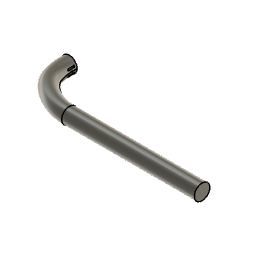
Base1 v7 (Autodesk Fusion 360 archive; units mm, degrees)
design "base pipe"
Autodesk Fusion 360 part; units mm, degrees
note: some values were not read from the file. Set by a fixed rule: which face or edge a step refers to.
sketch "Sketch1" plane through (0, 0, 0) normal (0, 0, 1) x (1, 0, 0)
  line L0 (100, 0) -> (50, 0)
  line L1 (50, 0) -> (20, 30)
  line L2 (20, 30) -> (10, 40)
  line L3 (10, 40) -> (0, 50)
  line L4 (0, 50) -> (0, 100)
  spline S0 degree 5 poles (100, 0) (50, 0) (20, 30) (10, 40) (0, 50) (0, 100) knots 0 0 0 0 0 0 1 1 1 1 1 1
pipe "Pipe1" add diameter 35 path "Sketch1" along S0
sketch "Sketch2" plane through (0, 0, 0) normal (0, 0, 1) x (1, 0, 0)
  line L0 (100, 0) -> (400, 0)
  dimension "d5" = 300
  constraint horizontal L0
  measures "d5" distance of L0.start L0.end
pipe "Pipe2" add diameter 35 path "Sketch2" along L0
sketch "Sketch3" plane through (0, 0, 0) normal (1, 0, 0) x (0, 1, 0)
sketch "Sketch4" plane through (0, 0, 0) normal (1, 0, 0) x (0, 1, 0)
  line L0 (80, -5.1) -> (80, -8.1)
  line L1 (80, -8.1) -> (95.5, -8.1)
  line L2 (95.5, 8.1) -> (80, 8.1)
  line L3 (80, 8.1) -> (80, 5.1)
  line L4 (80, 5.1) -> (95.5, 5.1)
  line L5 (80, -8.1) -> (80, -5.1)
  line L6 (80, -5.1) -> (95.5, -5.1)
  line L7 (80, 8.1) -> (80, 5.1)
  line L8 (80, -5.1) -> (80, -8.1)
  line L9 (95.5, -8.1) -> (95.5, -5.1)
  line L10 (95.5, 5.1) -> (95.5, 8.1)
  circle A0 centre (87.75, -0.0648) radius 1.5
  dimension "d15" = 15.5
  dimension "d16" = 16.2
  dimension "d17" = 3
  dimension "d18" = 3
  dimension "d19" = 3
  constraint vertical L0
  constraint horizontal L1
  constraint vertical L9
  constraint horizontal L2
  constraint vertical L7
  constraint vertical L3
  constraint coincident L4.end L9
  constraint perpendicular L4 L9
  constraint coincident L0.start L7
  constraint perpendicular L6 L9
  constraint collinear L7 L8
  constraint collinear L9 L10
  measures "d15" distance of L0.end L1.end
  measures "d16" distance of L0.end L2.end
  measures "d17" distance of L2.end L3.end
  measures "d18" distance of L0.end L0.start
  measures "d19" diameter of A0
extrude "Extrude1" cut sketch "Sketch4" along normal blind 40
extrude "Extrude2" add 1 faces at (0, 90.3333, 6.1) along direction (1, 0, 0) blind 12.5

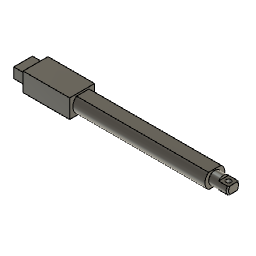
design "LINEAR-ACTUATOR"
Autodesk Fusion 360 part; units mm, degrees
sketch "Sketch1" plane through (0, 0, 0) normal (0, 0, 1) x (1, 0, 0)
  line L0 (0, 0) -> (37.4, 0)
  line L1 (37.4, 0) -> (37.4, 20)
  line L2 (37.4, 20) -> (0, 20)
  line L3 (0, 20) -> (0, 0)
  dimension "d1" = 37.4
  dimension "d2" = 20
  constraint horizontal L0
  constraint vertical L1
  constraint horizontal L2
  constraint vertical L3
  constraint coincident L0.start L3.end
  measures "d1" distance of L0.start L0.end
  measures "d2" distance of L0.start L2.end
extrude "Extrude1" add sketch "Sketch1" along normal blind 15
sketch "Sketch2" plane through (37.4, 0, 0) normal (1, 0, 0) x (0, 1, 0)
  line L0 (0, 0) -> (20, 0)
  line L1 (20, 0) -> (20, 15)
  line L2 (20, 15) -> (0, 15)
  line L3 (0, 15) -> (0, 0)
  line L4 (2.5, 13.5) -> (18.5, 13.5)
  line L5 (18.5, 13.5) -> (18.5, 1.5)
  line L6 (18.5, 1.5) -> (2.5, 1.5)
  line L7 (2.5, 1.5) -> (2.5, 13.5)
  line L8 (2.5, 13.5) -> (5.5, 13.5)
  line L9 (2.5, 1.5) -> (5.5, 1.5)
  arc A0 (5.5, 13.5) -> (5.5, 1.5) centre (10, 7.5) ccw
  line L10 (10.5, 13.5) -> (10.5, 1.5)
  arc A1 (15.5, 1.5) -> (15.5, 13.5) centre (11, 7.5) ccw
  dimension "d5" = 16
  dimension "d6" = 12
  dimension "d7" = 1.5
  dimension "d8" = 1.5
  dimension "d9" = 3
  dimension "d10" = 3
  dimension "d23" = 10
  constraint horizontal L4
  constraint vertical L5
  constraint horizontal L6
  constraint vertical L7
  constraint perpendicular L7 L8
  constraint perpendicular L7 L9
  constraint midpoint L4 L10.start
  constraint midpoint L6 L10.end
  constraint symmetric L8.end L10 A1.end
  constraint symmetric L9.end L10 A1.start
  constraint symmetric A0 L10 A1
  constraint tangent L7 A0
  measures "d5" distance of L4.start L4.end
  measures "d6" distance of L4.start L6.end
  measures "d7" distance of L1 L5
  measures "d8" distance of L2 L4
  measures "d9" distance of L4.start L8.end
  measures "d10" distance of L6.end L9.end
  measures "d23" distance of L8.end A1.end
extrude "Extrude2" add sketch "Sketch2" along normal blind 106 contours L4 L6 A0 L10 | L4 L6 L10 A1
sketch "Sketch3" plane through (0, 0, 0) normal (-1, 0, 0) x (0, -1, 0)
  line L0 (-20, 0) -> (0, 0)
  line L1 (0, 0) -> (0, 15)
  line L2 (0, 15) -> (-20, 15)
  line L3 (-20, 15) -> (-20, 0)
  line L4 (-2.5, 3.5) -> (-17.5, 3.5)
  line L5 (-17.5, 3.5) -> (-17.5, 11.6)
  line L6 (-17.5, 11.6) -> (-2.5, 11.6)
  line L7 (-2.5, 11.6) -> (-2.5, 3.5)
  line L8 (-10, 0) -> (-10, 15)
  line L9 (-20, 7.5) -> (0, 7.5)
  dimension "d13" = 15
  dimension "d14" = 8.1
  dimension "d15" = 4
  dimension "d16" = 7.5
  constraint horizontal L4
  constraint vertical L5
  constraint horizontal L6
  constraint vertical L7
  constraint midpoint L0 L8.start
  constraint midpoint L2 L8.end
  constraint midpoint L3 L9.start
  constraint midpoint L1 L9.end
  measures "d13" distance of L4.start L4.end
  measures "d14" distance of L4.end L5.end
  measures "d15" distance of L4 L9
  measures "d16" distance of L7 L8
extrude "Extrude3" add sketch "Sketch3" along normal blind 10 contours L4 L7 L8 L9 | L4 L5 L8 L9 | L5 L6 L8 L9 | L6 L7 L8 L9
fillet "Fillet1" [suppressed]
fillet "Fillet2" [suppressed]
sketch "Sketch4" plane through (143.4, 0, 0) normal (1, 0, 0) x (0, 1, 0)
  arc A0 (5.5, 13.5) -> (5.5, 1.5) centre (10, 7.5) ccw
  line L0 (5.5, 1.5) -> (15.5, 1.5)
  arc A1 (15.5, 1.5) -> (15.5, 13.5) centre (11, 7.5) ccw
  line L1 (15.5, 13.5) -> (5.5, 13.5)
  line L2 (5.5, 13.5) -> (15.5, 1.5)
  circle A2 centre (10.5, 7.5) radius 5
  dimension "d24" = 10
  constraint coincident A0.start L1.end
  constraint coincident L0.end A1.start
  constraint midpoint L2 A2.centre
  measures "d24" diameter of A2
extrude "Extrude4" add sketch "Sketch4" along normal blind 7 contours L2 A2 | L2 A2
sketch "Sketch5" plane through (150.4, 0, 0) normal (1, 0, 0) x (0, 1, 0)
  circle A0 centre (10.5, 7.5) radius 5
  line L0 (10.5, 7.5) -> (15.5, 7.5)
  line L1 (14.5, 10.5) -> (6.5, 10.5)
  line L2 (14.5, 4.5) -> (6.5, 4.5)
  dimension "d27" = 3
  constraint coincident A0.centre L0.start
  constraint coincident A0 L0.end
  constraint horizontal L0
  constraint coincident A0 L1.start
  constraint coincident A0 L1.end
  constraint horizontal L1
  constraint symmetric L0 L1.start L2.start
  constraint symmetric L0 L1.end L2.end
  measures "d27" distance of L0 L1
extrude "Extrude5" add sketch "Sketch5" along normal blind 8 contours A0 L1 L2
sketch "Sketch6" plane through (0, 0, 4.5) normal (0, 0, -1) x (1, 0, 0)
  line L0 (150.4, -6.5) -> (150.4, -14.5)
  line L1 (150.4, -14.5) -> (158.4, -14.5)
  line L2 (158.4, -14.5) -> (158.4, -6.5)
  line L3 (158.4, -6.5) -> (150.4, -6.5)
  line L4 (158.4, -6.5) -> (150.4, -14.5)
  circle A0 centre (154.4, -10.5) radius 2
  dimension "d30" = 4
  constraint coincident L2.end L3.start
  constraint coincident L0.end L1.start
  constraint midpoint L4 A0.centre
  measures "d30" diameter of A0
extrude "Extrude6" cut sketch "Sketch6" against normal blind 9 contours L4 A0 | L4 A0
fillet "Fillet3" radius 1 2 edges at (158.4, 5.5, 7.5) (158.4, 15.5, 7.5)
equation "d10 = d9"

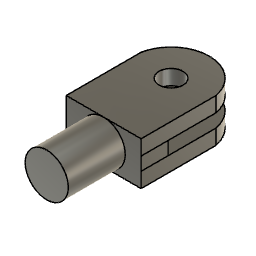
design "lever attach"
Autodesk Fusion 360 part; units mm, degrees
sketch "Sketch1" plane through (0, 0, 0) normal (0, 0, 1) x (1, 0, 0)
  arc A0 (50, 25) -> (25, 25) centre (37.5, 22.5) ccw
  line L0 (0, 0) -> (75, 0)
  circle A1 centre (37.5, 22.5) radius 7.5
  line L1 (25, 25) -> (25, 0)
  line L2 (50, 25) -> (50, 0)
  dimension "d1" = 15
  constraint coincident L0.start origin
  constraint horizontal L0
  constraint concentric A0 A1
  constraint coincident L0 L1.end
  constraint perpendicular L0 L1
  constraint coincident L0 L2.end
  constraint perpendicular L0 L2
  measures "d1" diameter of A1
extrude "Extrude1" add sketch "Sketch1" along normal blind 5 makes body 1
copy_body "CopyPasteBodies1" bodies 1 makes body 2
move_body "Move1" bodies 2 to x (1, 0, 0) y (0, 1, 0) z (0, 0, 1) at (0, 0, 9.4)
sketch "Sketch2" plane through (0, 0, 0) normal (0, -1, 0) x (1, 0, 0)
  line L0 (25, 9.4) -> (50, 9.4)
  line L1 (50, 9.4) -> (50, 14.4)
  line L2 (50, 14.4) -> (25, 14.4)
  line L3 (25, 14.4) -> (25, 9.4)
  line L4 (25, 5) -> (25, 9.4)
  line L5 (50, 5) -> (50, 9.4)
  line L6 (25, 5) -> (50, 5)
  line L7 (50, 9.4) -> (25, 9.4)
  constraint coincident L0.start L3.end
  constraint coincident L0.end L1.start
  constraint parallel L0 L6
extrude "Extrude2" add sketch "Sketch2" against normal blind 9 contours L0 L4 L5 L6 L7 bodies 1 2
sketch "Sketch3" plane through (0, 0, 0) normal (0, -1, 0) x (1, 0, 0)
  line L0 (25, 0) -> (50, 0)
  line L1 (50, 0) -> (50, 5)
  line L2 (50, 5) -> (50, 9.4)
  line L3 (50, 9.4) -> (50, 14.4)
  line L4 (50, 14.4) -> (25, 14.4)
  line L5 (25, 14.4) -> (25, 9.4)
  line L6 (25, 9.4) -> (25, 5)
  line L7 (25, 5) -> (25, 0)
  circle A0 centre (37.5, 7.2) radius 7.2
  constraint tangent L0 A0
extrude "Extrude3" add sketch "Sketch3" along normal blind 19 contours A0 bodies 1
move_face "OffsetFaces1" offset 3.5 1 faces at (44.9907, 22.1262, 12.7333) on bodies 1
move_face "OffsetFaces2" offset 3.5 1 faces at (44.9907, 22.1262, 3.3333) on bodies 1

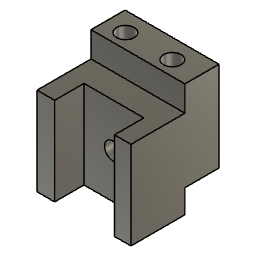
design "Midconnector"
Autodesk Fusion 360 part; units mm, degrees
sketch "Sketch1" plane through (0, 0, 0) normal (0, 0, 1) x (1, 0, 0)
  line L0 (16, 0) -> (16, 15)
  line L1 (16, 15) -> (0, 15)
  line L2 (0, 15) -> (0, 0)
  line L3 (0, 0) -> (3, 0)
  line L4 (3, 0) -> (3, 5)
  line L5 (3, 5) -> (13.2, 5)
  line L6 (13.2, 5) -> (13.2, 0)
  line L7 (0, 0) -> (3, 0)
  line L8 (13.2, 0) -> (16, 0)
  dimension "d1" = 16
  dimension "d2" = 15
  dimension "d3" = 5
  dimension "d4" = 10.2
  constraint horizontal L7
  constraint vertical L0
  constraint horizontal L1
  constraint vertical L2
  constraint coincident L2.end L3.start
  constraint perpendicular L4 L7
  constraint perpendicular L4 L5
  constraint coincident L6.end L7
  constraint perpendicular L6 L7
  constraint collinear L7 L8
  measures "d1" distance of L2.end L0.start
  measures "d2" distance of L2.end L1.end
  measures "d3" distance of L3.end L4.end
  measures "d4" distance of L4.end L5.end
extrude "Extrude1" add sketch "Sketch1" along normal blind 15
sketch "Sketch2" plane through (0, 5, 0) normal (0, -1, 0) x (1, 0, 0)
  line L0 (3, 0) -> (13.2, 0)
  line L1 (13.2, 0) -> (13.2, 15)
  line L2 (13.2, 15) -> (3, 15)
  line L3 (3, 15) -> (3, 0)
  line L4 (0, 0) -> (3, 0)
  line L5 (8, 6) -> (8, 7.5)
  circle A0 centre (8, 7.5) radius 1.5
  dimension "d9" = 3
  constraint coincident L4.start origin
  constraint parallel L0 L4
  constraint perpendicular L4 L5
  constraint coincident L5.end A0.centre
  constraint coincident A0 L5.start
  measures "d9" diameter of A0
extrude "Extrude2" cut sketch "Sketch2" against normal blind 19 contours A0
sketch "Sketch3" plane through (0, 15, 0) normal (0, 1, 0) x (-1, 0, 0)
  circle A0 centre (-8, 7.5) radius 1.5
  line L0 (-16, 0) -> (0, 0)
  line L1 (0, 0) -> (0, 15)
  line L2 (0, 15) -> (-16, 15)
  line L3 (-16, 15) -> (-16, 0)
  line L4 (0, 0) -> (0, 4)
  line L5 (0, 4) -> (-16, 4)
  line L6 (0, 15) -> (0, 11)
  line L7 (0, 11) -> (-16, 11)
  dimension "d12" = 4
  dimension "d13" = 4
  constraint coincident L0.end L1.start
  constraint perpendicular L0 L4
  constraint coincident L3 L5.end
  constraint perpendicular L3 L5
  constraint coincident L1.end L2.start
  constraint perpendicular L2 L6
  constraint coincident L3 L7.end
  constraint perpendicular L3 L7
  measures "d12" distance of L0.end L4.end
  measures "d13" distance of L1.end L6.end
extrude "Extrude3" cut sketch "Sketch3" against normal blind 5.8 contours L0 L1 L3 L4 L5 | L1 L2 L3 L6 L7
sketch "Sketch4" plane through (0, 0, 11) normal (0, 0, 1) x (-1, 0, 0)
  line L0 (-16, -15) -> (0, -15)
  line L1 (0, -15) -> (0, -9.2)
  line L2 (0, -9.2) -> (-16, -9.2)
  line L3 (-16, -9.2) -> (-16, -15)
  line L4 (-12.85, -11.7) -> (-11.35, -11.7)
  circle A0 centre (-11.35, -11.7) radius 1.5
  circle A1 centre (-3.35, -11.7) radius 1.5
  line L5 (-11.35, -11.7) -> (-9.85, -11.7)
  line L6 (-4.85, -11.7) -> (-3.35, -11.7)
  dimension "d18" = 3
  dimension "d19" = 8
  dimension "d20" = 3
  constraint coincident L4.end A0.centre
  constraint parallel L4 L5
  constraint coincident A1.centre L6.end
  constraint coincident A0 L5.end
  constraint coincident A1 L6.start
  constraint collinear L5 L6
  constraint coincident A0 L4.start
  measures "d18" diameter of A0
  measures "d19" distance of L4.end A1.centre
  measures "d20" diameter of A1
extrude "Extrude4" cut sketch "Sketch4" against normal blind 2 contours L4 A0 L5 | L4 A0 L5 | A1
sketch "Sketch5" plane through (0, 0, 4) normal (0, 0, -1) x (1, 0, 0)
  line L0 (0, -15) -> (16, -15)
  line L1 (16, -15) -> (16, -9.2)
  line L2 (16, -9.2) -> (0, -9.2)
  line L3 (0, -9.2) -> (0, -15)
  circle A0 centre (4.65, -11.7) radius 1.5
  circle A1 centre (12.65, -11.7) radius 1.5
  line L4 (11.15, -11.7) -> (12.65, -11.7)
  dimension "d25" = 3
  dimension "d26" = 8
  dimension "d27" = 3
  constraint coincident A1.centre L4.end
  constraint coincident A1 L4.start
  measures "d25" diameter of A0
  measures "d26" distance of A0.centre A1.centre
  measures "d27" diameter of A1
extrude "Extrude5" cut sketch "Sketch5" against normal blind 2 contours A0 | A1
move_face "OffsetFaces1" offset 8.325 1 faces at (14.9444, 12.0412, 11)

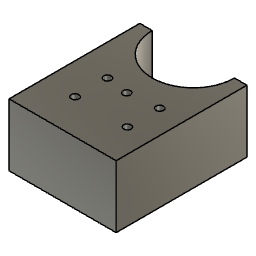
design "Torch holder connector1"
Autodesk Fusion 360 part; units mm, degrees
sketch "Sketch1" plane through (0, 0, 0) normal (0, 0, 1) x (1, 0, 0)
  line L0 (0, 0) -> (43, 0)
  line L1 (43, 0) -> (43, 52.5)
  line L2 (0, 52.5) -> (0, 0)
  arc A0 (5, 52.5) -> (38, 52.5) centre (21.5, 52.5) ccw
  line L3 (43, 52.5) -> (38, 52.5)
  line L4 (5, 52.5) -> (0, 52.5)
  line L5 (11, 14) -> (12.5, 14)
  circle A1 centre (12.5, 14) radius 1.5
  circle A2 centre (33.5, 14) radius 1.5
  circle A3 centre (12.5, 27) radius 1.5
  circle A4 centre (33.5, 27) radius 1.5
  line L6 (33.5, 14) -> (33.5, 15.5)
  line L7 (33.5, 25.5) -> (33.5, 27)
  line L8 (12.5, 14) -> (14, 14)
  line L9 (32, 14) -> (33.5, 14)
  line L10 (12.5, 14) -> (12.5, 15.5)
  line L11 (12.5, 25.5) -> (12.5, 27)
  line L12 (21.5, 28.25) -> (21.5, 26.75)
  line L13 (21.5, 0) -> (21.5, 25.75)
  circle A5 centre (21.5, 25.75) radius 1.5
  dimension "d1" = 43
  dimension "d2" = 52.5
  dimension "d6" = 3
  dimension "d7" = 21
  dimension "d8" = 3
  dimension "d9" = 13
  dimension "d10" = 3
  dimension "d11" = 13
  dimension "d12" = 3
  dimension "d15" = 25.75
  dimension "d16" = 3
  constraint horizontal L0
  constraint vertical L1
  constraint horizontal L3
  constraint vertical L2
  constraint coincident L0.start L2.end
  constraint coincident A0.start L3
  constraint collinear L3 L4
  constraint coincident A0.centre L3
  constraint coincident L5.end A1.centre
  constraint coincident A1 L5.start
  constraint parallel L5 L8
  constraint coincident A2.centre L6.start
  constraint perpendicular L5 L10
  constraint coincident A3.centre L11.end
  constraint perpendicular L6 L8
  constraint coincident A4.centre L7.end
  constraint coincident A2 L6.end
  constraint coincident A4 L7.start
  constraint collinear L6 L7
  constraint coincident A1 L8.end
  constraint coincident A2 L9.start
  constraint collinear L8 L9
  constraint coincident A1 L10.end
  constraint coincident A3 L11.start
  constraint collinear L10 L11
  constraint vertical L12
  constraint midpoint L0 L13.start
  constraint perpendicular L0 L13
  constraint coincident L13.end A5.centre
  measures "d1" distance of L0.start L0.end
  measures "d2" distance of L0.start L2.start
  measures "d6" diameter of A1
  measures "d7" distance of L5.end A2.centre
  measures "d8" diameter of A2
  measures "d9" distance of L5.end A3.centre
  measures "d10" diameter of A3
  measures "d11" distance of A2.centre A4.centre
  measures "d12" diameter of A4
  measures "d15" distance of L13.start L13.end
  measures "d16" diameter of A5
extrude "Extrude1" add sketch "Sketch1" along normal blind 25

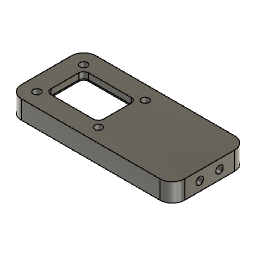
design "ACTUATOR-SLIDER-TOP-CONNECTOR"
Autodesk Fusion 360 part; units mm, degrees
sketch "Sketch1" plane through (0, 0, 0) normal (0, 0, 1) x (1, 0, 0)
  line L0 (2, 0) -> (28.3, 0)
  line L1 (30.3, 2) -> (30.3, 22.3)
  line L2 (28.3, 24.3) -> (2, 24.3)
  line L3 (0, 22.3) -> (0, 2)
  arc A0 (0, 2) -> (2, 0) centre (2, 2) ccw
  arc A1 (2, 24.3) -> (0, 22.3) centre (2, 22.3) ccw
  arc A2 (30.3, 22.3) -> (28.3, 24.3) centre (28.3, 22.3) ccw
  arc A3 (28.3, 0) -> (30.3, 2) centre (28.3, 2) ccw
  line L4 (-3, 22.3) -> (-3, 2)
  arc A4 (-3, 2) -> (2, -3) centre (2, 2) ccw
  line L5 (2, -3) -> (28.3, -3)
  arc A5 (28.3, -3) -> (33.3, 2) centre (28.3, 2) ccw
  line L6 (33.3, 2) -> (33.3, 22.3)
  arc A6 (33.3, 22.3) -> (28.3, 27.3) centre (28.3, 22.3) ccw
  line L7 (28.3, 27.3) -> (2, 27.3)
  arc A7 (2, 27.3) -> (-3, 22.3) centre (2, 22.3) ccw
  line L8 (28.3, -3) -> (53.3, -3)
  line L9 (58.3, 2) -> (58.3, 22.3)
  line L10 (53.3, 27.3) -> (28.3, 27.3)
  line L11 (28.3, 27.3) -> (28.3, -3)
  arc A8 (58.3, 22.3) -> (53.3, 27.3) centre (53.3, 22.3) ccw
  arc A9 (53.3, -3) -> (58.3, 2) centre (53.3, 2) ccw
  point P0 (30.3, 0)
  point P1 (0, 24.3)
  point P2 (58.3, -3)
  dimension "d1" = 30.3
  dimension "d2" = 24.3
  dimension "d3" = 2
  dimension "d4" = 3
  dimension "d40" = 30
  dimension "d76" = 5
  dimension "d77" = 5
  constraint horizontal L0
  constraint vertical L1
  constraint horizontal L2
  constraint vertical L3
  constraint coincident origin L3
  constraint coincident origin L0
  constraint tangent L3 A0
  constraint tangent L0 A0
  constraint coincident P1 L3
  constraint coincident P1 L2
  constraint tangent L3 A1
  constraint tangent L2 A1
  constraint equal A0 A1
  constraint tangent L2 A2
  constraint tangent L1 A2
  constraint equal A0 A2
  constraint coincident P0 L1
  constraint coincident P0 L0
  constraint tangent L1 A3
  constraint tangent L0 A3
  constraint equal A0 A3
  constraint horizontal L8
  constraint vertical L9
  constraint horizontal L10
  constraint vertical L11
  constraint tangent L9 A8
  constraint tangent L10 A8
  constraint coincident P2 L8
  constraint coincident P2 L9
  constraint tangent L8 A9
  constraint tangent L9 A9
  measures "d1" distance of origin P0
  measures "d2" distance of origin P1
  measures "d3" radius of A0
  measures "d40" distance of L5.end P2
  measures "d76" radius of A8
  measures "d77" radius of A9
extrude "Extrude1" add sketch "Sketch1" along normal blind 5 contours L0 L2 L3 A0 A1 L4 A4 L5 L7 A7 L11 | L1 A2 A3 A5 L6 A6 L11
sketch "Sketch2" plane through (0, 0, 5) normal (0, 0, 1) x (-1, 0, 0)
  arc A0 (-28.3, 0) -> (-30.3, -2) centre (-28.3, -2) ccw
  line L0 (-28.3, 0) -> (-2, 0)
  arc A1 (0, -2) -> (-2, 0) centre (-2, -2) ccw
  line L1 (0, -2) -> (0, -22.3)
  arc A2 (-2, -24.3) -> (0, -22.3) centre (-2, -22.3) ccw
  line L2 (-2, -24.3) -> (-28.3, -24.3)
  arc A3 (-30.3, -22.3) -> (-28.3, -24.3) centre (-28.3, -22.3) ccw
  line L3 (-30.3, -22.3) -> (-30.3, -2)
  arc A4 (-2, -27.3) -> (3, -22.3) centre (-2, -22.3) ccw
  line L4 (3, -22.3) -> (3, -2)
  arc A5 (3, -2) -> (-2, 3) centre (-2, -2) ccw
  line L5 (-2, 3) -> (-28.3, 3)
  arc A6 (-28.3, 3) -> (-33.3, -2) centre (-28.3, -2) ccw
  line L6 (-33.3, -2) -> (-33.3, -22.3)
  arc A7 (-33.3, -22.3) -> (-28.3, -27.3) centre (-28.3, -22.3) ccw
  line L7 (-28.3, -27.3) -> (-2, -27.3)
  line L8 (-28.3, 3) -> (-58.3, 3)
  line L9 (-63.3, -2) -> (-63.3, -22.3)
  line L10 (-58.3, -27.3) -> (-28.3, -27.3)
  line L11 (-28.3, -27.3) -> (-28.3, 3)
  line L12 (-15.15, 3) -> (-15.15, -27.3)
  line L13 (3, -12.15) -> (-33.3, -12.15)
  line L14 (-2.65, -2.65) -> (-27.65, -2.65)
  line L15 (-27.65, -2.65) -> (-27.65, -21.65)
  line L16 (-27.65, -21.65) -> (-2.65, -21.65)
  line L17 (-2.65, -21.65) -> (-2.65, -2.65)
  line L18 (-15.15, -2.65) -> (-15.15, -21.65)
  line L19 (-2.65, -12.15) -> (-27.65, -12.15)
  circle A8 centre (-2.65, -2.65) radius 1.5
  circle A9 centre (-27.65, -2.65) radius 1.5
  circle A10 centre (-2.65, -21.65) radius 1.5
  circle A11 centre (-27.65, -21.65) radius 1.5
  line L20 (-23.8, -4.5) -> (-6.5, -4.5)
  line L21 (-25.8, -17.8) -> (-25.8, -6.5)
  line L22 (-6.5, -19.8) -> (-23.8, -19.8)
  line L23 (-4.5, -6.5) -> (-4.5, -17.8)
  arc A12 (-4.5, -6.5) -> (-6.5, -4.5) centre (-6.5, -6.5) ccw
  arc A13 (-23.8, -4.5) -> (-25.8, -6.5) centre (-23.8, -6.5) ccw
  arc A14 (-25.8, -17.8) -> (-23.8, -19.8) centre (-23.8, -17.8) ccw
  arc A15 (-6.5, -19.8) -> (-4.5, -17.8) centre (-6.5, -17.8) ccw
  arc A16 (-63.3, -22.3) -> (-58.3, -27.3) centre (-58.3, -22.3) ccw
  arc A17 (-58.3, 3) -> (-63.3, -2) centre (-58.3, -2) ccw
  point P0 (-63.3, 3)
  dimension "d9" = 35
  dimension "d34" = 25
  dimension "d35" = 19
  dimension "d36" = 3
  dimension "d37" = 3
  dimension "d38" = 3
  dimension "d39" = 3
  dimension "d54" = 2
  dimension "d75" = 0.65
  dimension "d78" = 5
  constraint horizontal L8
  constraint vertical L9
  constraint horizontal L10
  constraint vertical L11
  constraint coincident L5.end A6.start
  constraint coincident A7.end L7.start
  constraint midpoint L5 L12.start
  constraint midpoint L7 L12.end
  constraint midpoint L4 L13.start
  constraint midpoint L6 L13.end
  constraint horizontal L14
  constraint vertical L15
  constraint horizontal L16
  constraint vertical L17
  constraint midpoint L14 L18.start
  constraint midpoint L16 L18.end
  constraint midpoint L17 L19.start
  constraint midpoint L15 L19.end
  constraint collinear L12 L18
  constraint collinear L13 L19
  constraint coincident L14.start L17.end
  constraint coincident L14.end L15.start
  constraint coincident L16.end L17.start
  constraint coincident L15.end L16.start
  constraint parallel L0 L20
  constraint parallel L3 L21
  constraint parallel L2 L22
  constraint parallel L1 L23
  constraint tangent L20 A12
  constraint tangent L23 A12
  constraint tangent L20 A13
  constraint tangent L21 A13
  constraint equal A12 A13
  constraint tangent L21 A14
  constraint tangent L22 A14
  constraint equal A12 A14
  constraint tangent L22 A15
  constraint tangent L23 A15
  constraint equal A12 A15
  constraint tangent L10 A16
  constraint tangent L9 A16
  constraint coincident P0 L9
  constraint coincident P0 L8
  constraint tangent L9 A17
  constraint tangent L8 A17
  constraint equal A16 A17
  measures "d9" distance of L5.end P0
  measures "d34" distance of L14.start L14.end
  measures "d35" distance of L14.start L16.end
  measures "d36" diameter of A8
  measures "d37" diameter of A9
  measures "d38" diameter of A10
  measures "d39" diameter of A11
  measures "d54" radius of A12
  measures "d75" distance of L11 L15.end
  measures "d78" radius of A16
extrude "Extrude2" add sketch "Sketch2" along normal blind 2.5 contours A0 L3 L11 L13 A9 | L0 L5 L11 L12 | A0 L3 A6 L6 L11 L13 | L0 L11 L12 L14 A9 | L0 A1 L1 L4 A5 L5 L12 L13 | L0 A1 L1 L12 L13 L14 L17 A8 | A6 L6 A7 L8 L9 L10 A16 A17 | A3 L3 L11 L13 A11 | A3 L3 L6 A7 L11 L13 | L12 L13 L14 L17 L18 L19 A8 L20 L23 A12 | L12 L13 L14 L15 L18 L19 A9 L20 L21 A13 | L11 L13 L15 A9 | L11 L13 L15 A11 | L2 L11 L12 L16 A11 | L2 L7 L11 L12 | L12 L13 L15 L16 L18 L19 A11 L21 L22 A14 | L1 A2 L2 A4 L4 L7 L12 L13 | L1 A2 L2 L12 L13 L16 L17 A10 | L12 L13 L16 L17 L18 L19 A10 L22 L23 A15
sketch "Sketch3" plane through (0, 0, 5) normal (0, 0, -1) x (1, 0, 0)
  arc A0 (28.3, -27.3) -> (33.3, -22.3) centre (28.3, -22.3) ccw
  line L0 (28.3, -27.3) -> (58.3, -27.3)
  line L1 (63.3, -22.3) -> (63.3, -2)
  line L2 (58.3, 3) -> (28.3, 3)
  arc A1 (33.3, -2) -> (28.3, 3) centre (28.3, -2) ccw
  line L3 (33.3, -2) -> (33.3, -22.3)
  line L4 (58.3, -27.3) -> (53.3, -27.3)
  line L5 (53.3, -27.3) -> (53.3, 7)
  line L6 (53.3, 7) -> (58.3, 7)
  line L7 (58.3, 7) -> (58.3, -27.3)
  arc A2 (58.3, -27.3) -> (63.3, -22.3) centre (58.3, -22.3) ccw
  arc A3 (63.3, -2) -> (58.3, 3) centre (58.3, -2) ccw
  dimension "d10" = 5
  constraint horizontal L4
  constraint vertical L5
  constraint horizontal L6
  constraint vertical L7
  constraint coincident L0.end L4.start
  measures "d10" distance of L0.end L4.end
extrude "Extrude3" add sketch "Sketch3" along normal blind 5 contours A0 L0 L2 A1 L3 L5 | L0 L2 L4 L5 L7 | L1 L7 A2 A3
sketch "Sketch4" plane through (63.3, 0, 0) normal (1, 0, 0) x (0, 1, 0)
  line L0 (2, 0) -> (22.3, 0)
  line L1 (2, 0) -> (22.3, 0)
  line L2 (22.3, 0) -> (22.3, 7.5)
  line L3 (22.3, 7.5) -> (2, 7.5)
  line L4 (2, 7.5) -> (2, 0)
  line L5 (2, 3.75) -> (22.3, 3.75)
  circle A0 centre (8.15, 3.75) radius 1.5
  line L6 (12.15, 7.5) -> (12.15, 0)
  circle A1 centre (16.15, 3.75) radius 1.5
  line L7 (22.3, 0) -> (22.3, 7.5)
  line L8 (22.3, 7.5) -> (2, 7.5)
  line L9 (2, 7.5) -> (2, 0)
  dimension "d14" = 3
  dimension "d15" = 4
  constraint horizontal L1
  constraint vertical L2
  constraint horizontal L3
  constraint vertical L4
  constraint coincident L0.start L1.start
  constraint midpoint L4 L5.start
  constraint midpoint L2 L5.end
  constraint coincident L5 A0.centre
  constraint midpoint L3 L6.start
  constraint midpoint L0 L6.end
  constraint symmetric A0 L6 A1
  measures "d14" diameter of A0
  measures "d15" distance of A0.centre L6
extrude "Extrude4" cut sketch "Sketch4" against normal blind 20 contours L5 A0 | L5 A0 | L5 A1 | L5 A1
fillet "Fillet3" [rolled back] radius 7
sketch "Sketch5" plane through (0, 0, 7.5) normal (0, 0, 1) x (-1, 0, 0)
  arc A0 (-66.3, 7) -> (-73.3, 0) centre (-66.3, 0) ccw
  line L0 (-73.3, 0) -> (-73.3, -24.3)
  arc A1 (-73.3, -24.3) -> (-66.3, -31.3) centre (-66.3, -24.3) ccw
  line L1 (-66.3, -31.3) -> (-2, -31.3)
  arc A2 (-2, -31.3) -> (7, -22.3) centre (-2, -22.3) ccw
  line L2 (7, -22.3) -> (7, -2)
  arc A3 (7, -2) -> (-2, 7) centre (-2, -2) ccw
  line L3 (-2, 7) -> (-66.3, 7)
  circle A4 centre (-27.65, -2.65) radius 1.5
  circle A5 centre (-2.65, -2.65) radius 1.5
  circle A6 centre (-27.65, -21.65) radius 1.5
  circle A7 centre (-2.65, -21.65) radius 1.5
  line L4 (-63, -27.3) -> (-68.3, -27.3)
  line L5 (-68.3, -27.3) -> (-68.3, 3)
  line L6 (-68.3, 3) -> (-63, 3)
  line L7 (-63, 3) -> (-63, -27.3)
  line L8 (-73.3, -12.15) -> (7, -12.15)
  line L9 (-63, -12.15) -> (-68.3, -12.15)
  arc A8 (-25.8, -17.8) -> (-23.8, -19.8) centre (-23.8, -17.8) ccw
  line L10 (-25.8, -17.8) -> (-25.8, -6.5)
  arc A9 (-23.8, -4.5) -> (-25.8, -6.5) centre (-23.8, -6.5) ccw
  line L11 (-23.8, -4.5) -> (-6.5, -4.5)
  arc A10 (-4.5, -6.5) -> (-6.5, -4.5) centre (-6.5, -6.5) ccw
  line L12 (-4.5, -6.5) -> (-4.5, -17.8)
  arc A11 (-6.5, -19.8) -> (-4.5, -17.8) centre (-6.5, -17.8) ccw
  line L13 (-6.5, -19.8) -> (-23.8, -19.8)
  dimension "d48" = 5.3
  dimension "d49" = 30.3
  dimension "d50" = 5
  constraint horizontal L4
  constraint vertical L5
  constraint horizontal L6
  constraint vertical L7
  constraint midpoint L0 L8.start
  constraint midpoint L2 L8.end
  constraint midpoint L7 L9.start
  constraint midpoint L5 L9.end
  constraint collinear L8 L9
  measures "d48" distance of L4.start L4.end
  measures "d49" distance of L4.start L6.end
  measures "d50" distance of L0 L5
extrude "Extrude5" [rolled back] along distance -7.5 taper angle 0
fillet "Fillet4" [rolled back] radius 2.5
ref_plane "WorkPlane1" through (33.15, 12.15, -2.5) normal (0, 0, -1) x (-1, 0, 0)
mirror "Mirror1" [rolled back] mirror stitch tolerance 0.1
sketch "Sketch6" plane through (0, 0, -10) normal (0, 0, 1) x (-1, 0, 0)
  line L0 (-30.3, -2) -> (-30.3, -22.3)
  arc A0 (-30.3, -22.3) -> (-28.3, -24.3) centre (-28.3, -22.3) ccw
  line L1 (-28.3, -24.3) -> (-2, -24.3)
  arc A1 (-2, -24.3) -> (0, -22.3) centre (-2, -22.3) ccw
  line L2 (0, -22.3) -> (0, -2)
  arc A2 (0, -2) -> (-2, 0) centre (-2, -2) ccw
  line L3 (-2, 0) -> (-28.3, 0)
  arc A3 (-28.3, 0) -> (-30.3, -2) centre (-28.3, -2) ccw
  circle A4 centre (-27.65, -21.65) radius 1.5
  circle A5 centre (-2.65, -21.65) radius 1.5
  circle A6 centre (-27.65, -2.65) radius 1.5
  arc A7 (-25.8, -17.8) -> (-23.8, -19.8) centre (-23.8, -17.8) ccw
  line L4 (-25.8, -17.8) -> (-25.8, -6.5)
  arc A8 (-23.8, -4.5) -> (-25.8, -6.5) centre (-23.8, -6.5) ccw
  line L5 (-23.8, -4.5) -> (-6.5, -4.5)
  arc A9 (-4.5, -6.5) -> (-6.5, -4.5) centre (-6.5, -6.5) ccw
  line L6 (-4.5, -6.5) -> (-4.5, -17.8)
  arc A10 (-6.5, -19.8) -> (-4.5, -17.8) centre (-6.5, -17.8) ccw
  line L7 (-6.5, -19.8) -> (-23.8, -19.8)
  circle A11 centre (-2.65, -2.65) radius 1.5
extrude "Extrude6" [rolled back] along distance -2.5 taper angle 0
sketch "Sketch8" plane through (0, 0, -5) normal (0, 0, 1) x (-1, 0, 0)
  line L0 (-68.3, -24.8) -> (-68.3, 0.5)
  arc A0 (-65.8, 3) -> (-68.3, 0.5) centre (-65.8, 0.5) ccw
  line L1 (-65.8, 3) -> (-65.5, 3)
  arc A1 (-63, 0.5) -> (-65.5, 3) centre (-65.5, 0.5) ccw
  line L2 (-63, 0.5) -> (-63, -24.8)
  arc A2 (-65.5, -27.3) -> (-63, -24.8) centre (-65.5, -24.8) ccw
  line L3 (-65.5, -27.3) -> (-65.8, -27.3)
  arc A3 (-68.3, -24.8) -> (-65.8, -27.3) centre (-65.8, -24.8) ccw
  arc A4 (-28.3, 0) -> (-30.3, -2) centre (-28.3, -2) ccw
  line L4 (-28.3, 0) -> (-2, 0)
  arc A5 (0, -2) -> (-2, 0) centre (-2, -2) ccw
  line L5 (0, -2) -> (0, -22.3)
  arc A6 (-2, -24.3) -> (0, -22.3) centre (-2, -22.3) ccw
  line L6 (-2, -24.3) -> (-28.3, -24.3)
  arc A7 (-30.3, -22.3) -> (-28.3, -24.3) centre (-28.3, -22.3) ccw
  line L7 (-30.3, -22.3) -> (-30.3, -2)
  arc A8 (-66.3, 7) -> (-73.3, 0) centre (-66.3, 0) ccw
  line L8 (-73.3, 0) -> (-73.3, -24.3)
  arc A9 (-73.3, -24.3) -> (-66.3, -31.3) centre (-66.3, -24.3) ccw
  line L9 (-66.3, -31.3) -> (-2, -31.3)
  arc A10 (-2, -31.3) -> (7, -22.3) centre (-2, -22.3) ccw
  line L10 (7, -22.3) -> (7, -2)
  arc A11 (7, -2) -> (-2, 7) centre (-2, -2) ccw
  line L11 (-2, 7) -> (-66.3, 7)
  line L12 (-71.3, 0) -> (-71.3, -24.3)
  arc A12 (-71.3, -24.3) -> (-66.3, -29.3) centre (-66.3, -24.3) ccw
  line L13 (-66.3, -29.3) -> (-2, -29.3)
  arc A13 (-2, -29.3) -> (5, -22.3) centre (-2, -22.3) ccw
  line L14 (5, -22.3) -> (5, -2)
  arc A14 (5, -2) -> (-2, 5) centre (-2, -2) ccw
  line L15 (-2, 5) -> (-66.3, 5)
  arc A15 (-66.3, 5) -> (-71.3, 0) centre (-66.3, 0) ccw
  arc A16 (-32.3, -22.3) -> (-28.3, -26.3) centre (-28.3, -22.3) ccw
  line L16 (-2, -26.3) -> (-28.3, -26.3)
  arc A17 (-2, -26.3) -> (2, -22.3) centre (-2, -22.3) ccw
  line L17 (2, -2) -> (2, -22.3)
  arc A18 (2, -2) -> (-2, 2) centre (-2, -2) ccw
  line L18 (-28.3, 2) -> (-2, 2)
  arc A19 (-28.3, 2) -> (-32.3, -2) centre (-28.3, -2) ccw
  line L19 (-32.3, -22.3) -> (-32.3, -2)
  line L20 (-65.8, 4) -> (-65.5, 4)
  arc A20 (-62, 0.5) -> (-65.5, 4) centre (-65.5, 0.5) ccw
  line L21 (-62, 0.5) -> (-62, -24.8)
  arc A21 (-65.5, -28.3) -> (-62, -24.8) centre (-65.5, -24.8) ccw
  line L22 (-65.5, -28.3) -> (-65.8, -28.3)
  arc A22 (-69.3, -24.8) -> (-65.8, -28.3) centre (-65.8, -24.8) ccw
  line L23 (-69.3, -24.8) -> (-69.3, 0.5)
  arc A23 (-65.8, 4) -> (-69.3, 0.5) centre (-65.8, 0.5) ccw
  dimension "d70" = -2
  dimension "d73" = -2
  dimension "d74" = 1
  measures "d73" distance of A7
extrude "Extrude8" [rolled back] side1offset 0 taper angle 0
sketch "Sketch7" plane through (0, 0, -10) normal (0, 0, 1) x (-1, 0, 0)
  line L0 (-53.3, -24.8) -> (-53.3, 0.5)
  arc A0 (-50.8, 3) -> (-53.3, 0.5) centre (-50.8, 0.5) ccw
  line L1 (-50.8, 3) -> (-50.5, 3)
  arc A1 (-48, 0.5) -> (-50.5, 3) centre (-50.5, 0.5) ccw
  line L2 (-48, 0.5) -> (-48, -24.8)
  arc A2 (-50.5, -27.3) -> (-48, -24.8) centre (-50.5, -24.8) ccw
  line L3 (-50.5, -27.3) -> (-50.8, -27.3)
  arc A3 (-53.3, -24.8) -> (-50.8, -27.3) centre (-50.8, -24.8) ccw
  arc A4 (-28.3, 0) -> (-30.3, -2) centre (-28.3, -2) ccw
  line L4 (-28.3, 0) -> (-2, 0)
  arc A5 (0, -2) -> (-2, 0) centre (-2, -2) ccw
  line L5 (0, -2) -> (0, -22.3)
  arc A6 (-2, -24.3) -> (0, -22.3) centre (-2, -22.3) ccw
  line L6 (-2, -24.3) -> (-28.3, -24.3)
  arc A7 (-30.3, -22.3) -> (-28.3, -24.3) centre (-28.3, -22.3) ccw
  line L7 (-30.3, -22.3) -> (-30.3, -2)
  arc A8 (-51.3, 7) -> (-58.3, 0) centre (-51.3, 0) ccw
  line L8 (-58.3, 0) -> (-58.3, -24.3)
  arc A9 (-58.3, -24.3) -> (-51.3, -31.3) centre (-51.3, -24.3) ccw
  line L9 (-51.3, -31.3) -> (-2, -31.3)
  arc A10 (-2, -31.3) -> (7, -22.3) centre (-2, -22.3) ccw
  line L10 (7, -22.3) -> (7, -2)
  arc A11 (7, -2) -> (-2, 7) centre (-2, -2) ccw
  line L11 (-2, 7) -> (-51.3, 7)
  line L12 (7, -12.15) -> (-58.3, -12.15)
  line L13 (-58.3, -4.65) -> (-53.3, -4.65)
  line L14 (-53.3, -4.65) -> (-53.3, -19.65)
  line L15 (-53.3, -19.65) -> (-58.3, -19.65)
  line L16 (-58.3, -19.65) -> (-58.3, -4.65)
  line L17 (-53.3, -12.15) -> (-58.3, -12.15)
  line L18 (-36.65, -19.65) -> (-41.65, -19.65)
  line L19 (-41.65, -19.65) -> (-41.65, -4.65)
  line L20 (-41.65, -4.65) -> (-36.65, -4.65)
  line L21 (-36.65, -4.65) -> (-36.65, -19.65)
  line L22 (-36.65, -12.15) -> (-41.65, -12.15)
  line L23 (-30.3, -12.15) -> (-48, -12.15)
  line L24 (-39.15, -12.15) -> (-39.15, -31.3)
  line L25 (-39.15, -19.65) -> (-39.15, -4.65)
  line L26 (6, -4.65) -> (1, -4.65)
  line L27 (1, -4.65) -> (1, -19.65)
  line L28 (1, -19.65) -> (6, -19.65)
  line L29 (6, -19.65) -> (6, -4.65)
  line L30 (6, -12.15) -> (1, -12.15)
  line L31 (7, -12.15) -> (1, -12.15)
  line L32 (3.5, -4.65) -> (3.5, -19.65)
  line L33 (0, -12.15) -> (7, -12.15)
  line L34 (3.5, -12.15) -> (3.5, -25)
  dimension "d60" = 15
  dimension "d61" = 15
  dimension "d62" = 5
  dimension "d63" = 15
  constraint midpoint L10 L12.start
  constraint midpoint L8 L12.end
  constraint horizontal L13
  constraint vertical L14
  constraint horizontal L15
  constraint vertical L16
  constraint coincident L0 L14.end
  constraint coincident L8 L13.start
  constraint midpoint L14 L17.start
  constraint perpendicular L0 L17
  constraint midpoint L16 L12.end
  constraint collinear L12 L17
  constraint horizontal L18
  constraint vertical L19
  constraint horizontal L20
  constraint vertical L21
  constraint midpoint L21 L22.start
  constraint midpoint L19 L22.end
  constraint collinear L12 L22
  constraint midpoint L7 L23.start
  constraint midpoint L2 L23.end
  constraint midpoint L23 L24.start
  constraint coincident L9 L24.end
  constraint perpendicular L9 L24
  constraint midpoint L18 L25.start
  constraint midpoint L20 L25.end
  constraint collinear L24 L25
  constraint horizontal L26
  constraint vertical L27
  constraint horizontal L28
  constraint vertical L29
  constraint midpoint L29 L30.start
  constraint midpoint L27 L30.end
  constraint collinear L12 L30
  constraint midpoint L26 L32.start
  constraint midpoint L28 L32.end
  constraint midpoint L5 L33.start
  constraint midpoint L33 L34.start
  constraint perpendicular L12 L34
  constraint collinear L32 L34
  measures "d60" distance of L13.start L15.end
  measures "d61" distance of L18.start L20.end
  measures "d62" distance of L26.start L26.end
  measures "d63" distance of L26.start L28.end
extrude "Extrude7" [suppressed]
fillet "Fillet5" [suppressed]
